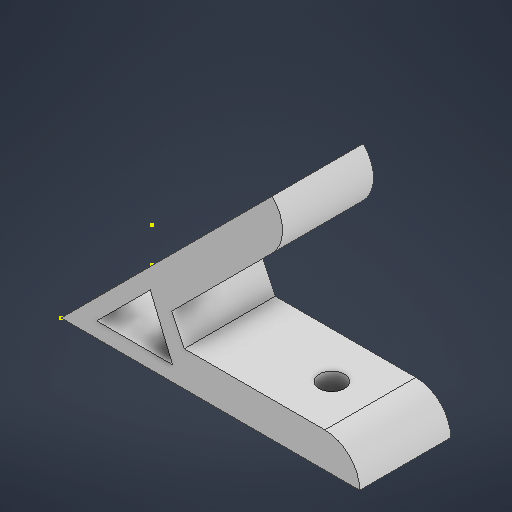
# Autodesk Inventor part: 45 Degree Connector
Saved by Autodesk Inventor 2026 (Build 300175050, 175E)
## iProperties
Created: 2025-07-01
Part Number: 45 Degree Connector
Material: Generic
Document SubType Name: Modeling
Designer: aadit
Density: 1 g/cm^3
Appearance: Default
Author: aadit
Autodesk Inventor part; units mm, degrees
ref_plane "YZ Plane" through (0, 0, 0) normal (1, 0, 0) x (0, 1, 0)
ref_plane "XZ Plane" through (0, 0, 0) normal (0, 1, 0) x (-1, 0, 0)
ref_plane "XY Plane" through (0, 0, 0) normal (0, 0, 1) x (1, 0, 0)
sketch "Sketch1" plane through (0, 0, 0) normal (0, 0, 1) x (1, 0, 0)
  line L0 (0, 0) -> (59, 0)
  line L1 (7, 3) -> (22, 3)
  line L2 (7, 3) -> (22, 3) construction
  line L3 (0, 0) -> (41.7193, 41.7193)
  line L4 (0, 0) -> (59, 0) construction
  line L5 (7, 3) -> (17.6066, 13.6066)
  line L6 (7, 3) -> (22, 3) construction
  line L7 (17.6066, 13.6066) -> (22, 3)
  line L8 (59, 0) -> (59, 6.89)
  line L9 (59, 6.89) -> (24, 6.89)
  line L10 (41.7193, 41.7193) -> (46.5913, 36.8473)
  line L11 (46.5913, 36.8473) -> (21.8425, 12.0986)
  line L12 (21.8425, 12.0986) -> (24.3232, 6.89)
  dimension "d0" = 59
  dimension "d1" = 15
  dimension "d3" = 59
  dimension "d4" = 45
  dimension "d5" = 15
  dimension "d6" = 45
  dimension "d7" = 6.89
  dimension "d8" = 35
  dimension "d10" = 6.89
  dimension "d11" = 35
  constraints: 26 end point, 4 horizontal, 3 equal length, 3 perpendicular, 1 parallel, 1 point on line
  measures "d0" distance of L0.start L0.end
  measures "d1" distance of L1.start L1.end
  measures "d3" distance of L0.start L3.end
  measures "d4" angle of L4 L3
  measures "d5" distance of L1.start L5.end
  measures "d6" angle of L6 L5
  measures "d7" distance of L4.end L8.end
  measures "d8" distance of L8.end L9.end
  measures "d10" distance of L3.end L10.end
  measures "d11" distance of L10.end L11.end
extrude "Extrusion1" add sketch "Sketch1" along normal blind 18
sketch "Sketch2" plane through (0, 0, 18) normal (0, 0, 1) x (1, 0, 0)
  point P0 (0, 0)
fillet "Fillet1" radius 6.89 1 edges at (46.5913, 36.8473, 9)
fillet "Fillet2" radius 6.89 1 edges at (59, 6.89, 9)
sketch "Sketch3" plane through (24.3232, 6.89, 18) normal (0, 1, 0) x (1, 0, 0)
  point P0 (-24.3232, 18)
sketch "Sketch4" plane through (0, 0, 0) normal (0, -1, 0) x (1, 0, 0)
  point P0 (0, 0)
sketch "Sketch5" plane through (0, 0, 0) normal (0, -1, 0) x (1, 0, 0)
  circle A0 centre (44.5, 9) radius 2.5
  point P0 (0, 0)
  dimension "d16" = 5
  constraints: 1 centre point
  measures "d16" diameter of A0
extrude "Extrusion2" cut sketch "Sketch5" against normal blind 6.89
sketch "Sketch6" plane through (0, 0, 0) normal (-0.7071, 0.7071, 0) x (-0.7071, -0.7071, 0)
  circle A0 centre (-44.5, 9) radius 2.5
  point P0 (0, 0)
  dimension "d19" = 5
  constraints: 1 centre point
  measures "d19" diameter of A0
extrude "Extrusion3" cut sketch "Sketch6" against normal blind 6.89
body "Solid1"
